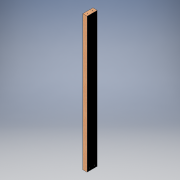
# Autodesk Inventor part: wallLeftShort
Saved by Autodesk Inventor 2016 (Build 200138000, 138)
## iProperties
Created: 2016-12-21
Part Number: wallLeftShort
Material: Wood (Birch)
Document SubType Name: Modeling
Designer: Naga
Density: 0.55 g/cm^3
Appearance: Birch - Natural Polished
Author: Naga
Autodesk Inventor part; units mm, degrees
ref_plane "YZ Plane" through (0, 0, 0) normal (1, 0, 0) x (0, 1, 0)
ref_plane "XZ Plane" through (0, 0, 0) normal (0, 1, 0) x (-1, 0, 0)
ref_plane "XY Plane" through (0, 0, 0) normal (0, 0, 1) x (1, 0, 0)
sketch "Sketch1" plane through (0, 0, 0) normal (0, 1, 0) x (-1, 0, 0)
  line L0 (0, 0) -> (38.1, 0)
  line L1 (38.1, 0) -> (38.1, -88.9)
  line L2 (38.1, -88.9) -> (0, -88.9)
  line L3 (0, -88.9) -> (0, 0)
  dimension "d0" = 38.1
  dimension "d1" = 88.9
  constraints: 8 end point, 2 parallel, 1 horizontal, 1 perpendicular
  measures "d0" distance of L1.end L2.end
  measures "d1" distance of L0.end L1.end
extrude "Wood" add sketch "Sketch1" along normal blind 1181.1
sketch "Sketch4" plane through (0, 1181.1, 0) normal (0, 1, 0) x (1, 0, 0)
  line L0 (-38.1, 0) -> (0, 0) projected
  line L1 (0, 88.9) -> (-38.1, 88.9) projected
  line L2 (0, 0) -> (-38.1, 0)
  line L3 (-38.1, 0) -> (-38.1, 88.9)
  line L4 (-38.1, 88.9) -> (0, 88.9)
  line L5 (0, 88.9) -> (0, 0)
  line L6 (-19.05, 88.9) -> (-38.1, 88.9)
  line L7 (-38.1, 88.9) -> (-38.1, 44.45)
  line L8 (-38.1, 44.45) -> (-19.05, 44.45)
  line L9 (-19.05, 44.45) -> (-19.05, 88.9)
  line L10 (-19.05, 66.675) -> (0, 66.675)
  line L11 (0, 66.675) -> (0, 44.45)
  line L12 (0, 44.45) -> (-19.05, 44.45)
  line L13 (-19.05, 44.45) -> (-19.05, 66.675)
  circle A0 centre (-19.05, 66.675) radius 2.3812
  circle A1 centre (-19.05, 22.225) radius 2.3812
  dimension "d11" = 4.7625
  constraints: 24 end point, 6 parallel, 4 midpoint, 3 horizontal, 3 perpendicular, 2 centre point, 1 coincident, 1 symmetric about line, 1 other
  measures "d11" diameter of A0
extrude "Extrusion4" cut sketch "Sketch4" against normal blind 38.1 contours A0 L9 | L9 L10 A0 | L10 L9 A0 | A1
sketch "Sketch5" plane through (0, 0, 0) normal (1, 0, 0) x (0, 0, -1)
  line L0 (88.9, 0) -> (0, 0) projected
  line L1 (88.9, 0) -> (88.9, 1181.1) projected
  line L2 (0, 0) -> (88.9, 0)
  line L3 (88.9, 0) -> (88.9, 38.1)
  line L4 (88.9, 38.1) -> (0, 38.1)
  line L5 (0, 38.1) -> (0, 0)
  line L6 (88.9, 0) -> (44.45, 0)
  line L7 (44.45, 0) -> (44.45, 38.1)
  line L8 (44.45, 38.1) -> (88.9, 38.1)
  line L9 (88.9, 38.1) -> (88.9, 0)
  line L10 (44.45, 38.1) -> (66.675, 38.1)
  line L11 (66.675, 38.1) -> (66.675, 19.05)
  line L12 (66.675, 19.05) -> (44.45, 19.05)
  line L13 (44.45, 19.05) -> (44.45, 38.1)
  circle A0 centre (66.675, 19.05) radius 2.3812
  circle A1 centre (22.225, 19.05) radius 2.3812
  dimension "d14" = 38.1
  dimension "d15" = 4.7625
  constraints: 24 end point, 6 parallel, 3 horizontal, 3 perpendicular, 2 centre point, 1 coincident, 1 midpoint, 1 point on line, 1 symmetric about line, 1 other
  measures "d14" distance of L3.end L2.end
  measures "d15" diameter of A0
extrude "Extrusion5" cut sketch "Sketch5" against normal up to surface (38.1 mm away) contours A0 L11 L12 | L12 L11 A0 | A1
body "Solid1"
